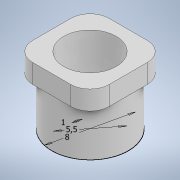
# Autodesk Inventor part: led
Saved by Autodesk Inventor 2021 (Build 250183000, 183)
## iProperties
Created: 2020-10-24
Part Number: led
Material: Générique
Document SubType Name: Modeling
Designer: sebas
Density: 1 g/cm^3
Appearance: Par défaut
Author: sebas
Autodesk Inventor part; units mm, degrees
ref_plane "YZ Plane" through (0, 0, 0) normal (1, 0, 0) x (0, 1, 0)
ref_plane "XZ Plane" through (0, 0, 0) normal (0, 1, 0) x (-1, 0, 0)
ref_plane "XY Plane" through (0, 0, 0) normal (0, 0, 1) x (1, 0, 0)
sketch "Esquisse1" plane through (0, 0, 0) normal (0, 1, 0) x (-1, 0, 0)
  circle A0 centre (0, 0) radius 4
  circle A1 centre (0, 0) radius 2.75
  line L0 (2.75, 0) -> (0, 0) construction
  circle A2 centre (1.375, 0) radius 0.5
  line L1 (0, 4) -> (0, -4)
  circle A3 centre (-1.375, 0) radius 0.5
  point P0 (0, 2.75)
  point P1 (0, -2.75)
  dimension "d1" = 5.5
  dimension "d0" = 8
  dimension "d2" = 1
  constraints: 4 end point, 3 centre point, 2 coincident, 2 point on circle, 1 horizontal, 1 midpoint, 1 symmetric about line, 1 vertical, 4 other
  measures "d0" diameter of A0
  measures "d2" diameter of A2
extrude "Extrusion1" add sketch "Esquisse1" along normal blind 2 contours L1 A1 | A1 L1
extrude "Extrusion2" add sketch "Esquisse1" along normal blind 7 contours A0 L1 A1 | L1 A1 A0
sketch "Esquisse2" plane through (0, 7, 0) normal (0, 1, 0) x (1, 0, 0)
  line L0 (4, 4) -> (-4, 4)
  line L1 (-4, 4) -> (-4, -4)
  line L2 (-4, -4) -> (4, -4)
  line L3 (4, -4) -> (4, 4)
  line L4 (4, 4) -> (-4, -4) construction
  line L5 (-4, 4) -> (4, -4) construction
  line L6 (-4, -4) -> (0, -4)
  circle A0 centre (0, 0) radius 4 projected
  line L7 (-4, 0) -> (-4, -4)
  arc A1 (-4, 0) -> (0, -4) centre (0, 0) ccw
  line L8 (-4, 0) -> (-4, 4)
  line L9 (0, 4) -> (-4, 4)
  arc A2 (0, 4) -> (-4, 0) centre (0, 0) ccw
  line L10 (0, -4) -> (4, -4)
  line L11 (4, -4) -> (4, 0)
  line L12 (4, 0) -> (4, 4)
  line L13 (4, 4) -> (0, 4)
  arc A3 (0, -4) -> (4, 0) centre (0, 0) ccw
  arc A4 (4, 0) -> (0, 4) centre (0, 0) ccw
  constraints: 28 end point, 12 point on circle, 7 tangent, 6 midpoint, 4 centre point, 3 perpendicular, 2 collinear, 2 parallel, 1 concentric, 1 horizontal
extrude "Extrusion3" add sketch "Esquisse2" against normal blind 2 contours L3 A0 L0 | A0 L1 L0 | L3 L2 A0 | A0 L2 L1
fillet "Congé1" radius 2 4 edges at (-4, 6, 4) (4, 6, 4) (4, 6, -4) (-4, 6, -4)
